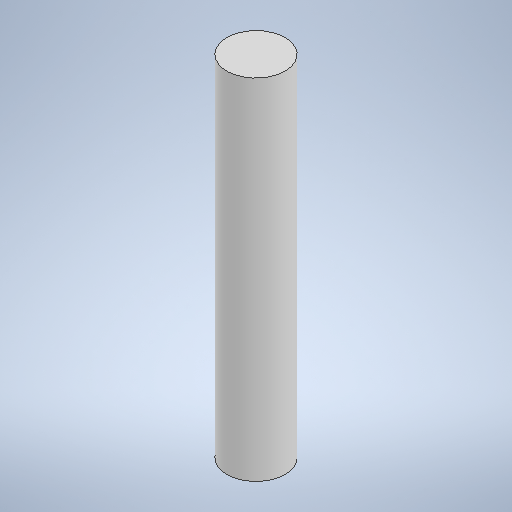
# Autodesk Inventor part: Index_Pin
Saved by Autodesk Inventor 2025 (Build 290162000, 162)
## iProperties
Created: 2026-07-08
Part Number: Index_Pin
Material: Generisch
Document SubType Name: Modeling
Designer: wavid
Mass: 0.301593 g
Surface Area: 3.26726 cm^2
Volume: 0.301593 cm^3
Density: 1 g/cm^3
Appearance: Vorgabe
Author: wavid
Autodesk Inventor part; units mm, degrees
ref_plane "YZ Plane" through (0, 0, 0) normal (1, 0, 0) x (0, 1, 0)
ref_plane "XZ Plane" through (0, 0, 0) normal (0, 1, 0) x (-1, 0, 0)
ref_plane "XY Plane" through (0, 0, 0) normal (0, 0, 1) x (1, 0, 0)
sketch "Skizze1" plane through (0, 0, 0) normal (0, 0, 1) x (1, 0, 0)
  circle A0 centre (0, 0) radius 2
  dimension "d0" = 24
  constraints: 1 centre point
extrude "Extrusion1" add sketch "Skizze1" along normal blind 24
